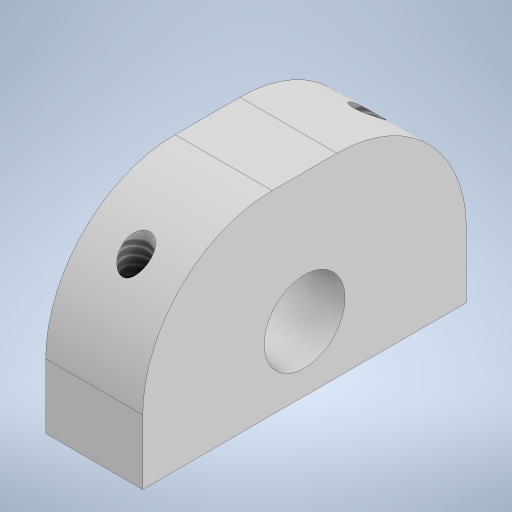
# Autodesk Inventor part: Lock Base
Saved by Autodesk Inventor 2023 (Build 270158000, 158)
## iProperties
Created: 2022-12-20
Part Number: Lock Base
Material: Generic
Document SubType Name: Modeling
Designer: Hayden Swanson
Density: 1 g/cm^3
Appearance: Default
Author: Hayden Swanson
Autodesk Inventor part; units mm, degrees
ref_plane "YZ Plane" through (0, 0, 0) normal (1, 0, 0) x (0, 1, 0)
ref_plane "XZ Plane" through (0, 0, 0) normal (0, 1, 0) x (-1, 0, 0)
ref_plane "XY Plane" through (0, 0, 0) normal (0, 0, 1) x (1, 0, 0)
sketch "Sketch1" plane through (0, 0, 0) normal (0, 1, 0) x (-1, 0, 0)
  line L0 (0, 0) -> (7.62, 0)
  line L1 (7.62, 0) -> (7.62, -25.4)
  line L2 (7.62, -25.4) -> (0, -25.4)
  line L3 (0, -25.4) -> (0, 0)
  dimension "d1" = 7.62
  dimension "d2" = 25.4
  constraints: 8 end point, 2 parallel, 1 horizontal, 1 perpendicular
  measures "d1" distance of L1.end L2.end
  measures "d2" distance of L0.end L1.end
extrude "Extrusion1" add sketch "Sketch1" along normal blind 15.24
sketch "Sketch2" plane through (-7.62, 0, -25.4) normal (-1, 0, 0) x (0, 0, 1)
  line L0 (0, 15.24) -> (25.4, 15.24) projected
  circle A0 centre (12.7, 5.08) radius 3.175
  line L1 (0, 0) -> (25.4, 0) projected
  line L2 (12.7, 5.08) -> (12.7, 0)
  line L3 (0, 0) -> (12.7, 0)
  line L4 (12.7, 0) -> (25.4, 0)
  dimension "d45" = 6.35
  dimension "d58" = 5.08
  constraints: 6 end point, 1 centre point, 1 collinear, 1 midpoint
  measures "d45" diameter of A0
  measures "d58" distance of L2.start L2.end
extrude "Extrusion2" cut sketch "Sketch2" against normal blind 17.78
sketch "Sketch3" plane through (0, 0, 0) normal (0, -1, 0) x (1, 0, 0)
  line L0 (-7.62, 0) -> (0, 0) projected
  line L1 (-3.81, 0) -> (-3.81, -2.54)
  line L2 (0, -25.4) -> (-7.62, -25.4) projected
  line L3 (-3.81, -25.4) -> (-3.81, -22.86)
  line L4 (-3.81, -2.54) -> (-3.81, -3.302)
  circle A0 centre (-3.81, -3.302) radius 1.4224
  line L5 (-3.81, -22.86) -> (-3.81, -21.4376)
  circle A1 centre (-3.81, -21.4376) radius 1.4224
  dimension "d46" = 2.8448
  dimension "d29" = 2.54
  dimension "d30" = 2.54
  dimension "d31" = 0.762
  dimension "d32" = 2.8448
  constraints: 8 end point, 4 vertical, 2 coincident, 2 midpoint, 1 centre point, 1 vertical alignment, 2 other
  measures "d29" distance of L1.start L1.end
  measures "d30" distance of L3.start L3.end
  measures "d31" distance of L1.end L4.end
  measures "d32" diameter of A0
fillet "Fillet1" radius 10.16 2 edges at (-3.81, 15.24, -25.4) (-3.81, 15.24, 0)
hole "Hole1" at (-3.81, 0, -3.302) at (-3.81, 0, -21.4376) direction (0, 1, 0) diameter 2.1565 end through all thread size "4-40 UNC" class "3B" standard "ANSI Unified Screw Threads"
body "Solid1"
